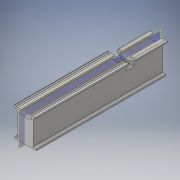
# Autodesk Inventor part: BED
Saved by Autodesk Inventor 2016 (Build 200138000, 138)
## iProperties
Created: 2017-02-14
Part Number: BED
Material: Generic
Document SubType Name: Modeling
Designer: M228540
Density: 1 g/cm^3
Appearance: Default
Author: M228540
Autodesk Inventor part; units mm, degrees
ref_plane "YZ Plane" through (0, 0, 0) normal (1, 0, 0) x (0, 1, 0)
ref_plane "XZ Plane" through (0, 0, 0) normal (0, 1, 0) x (-1, 0, 0)
ref_plane "XY Plane" through (0, 0, 0) normal (0, 0, 1) x (1, 0, 0)
sketch "Sketch1" plane through (0, 0, 0) normal (0, 0, 1) x (1, 0, 0)
  line L0 (11.5953, 6.0815) -> (2.069, 11.5815)
  line L1 (11.5953, 6.0815) -> (22.5953, 6.0815) construction
  line L2 (2.069, 11.5815) -> (-7.931, 11.5815)
  line L3 (-7.931, 11.5815) -> (-7.931, 23.2815)
  line L4 (-7.931, 23.2815) -> (0.1681, 32.9336)
  line L5 (0.1681, 32.9336) -> (3.9681, 32.9336)
  line L6 (3.9681, 32.9336) -> (11.7818, 26.3772)
  line L7 (11.7818, 26.3772) -> (11.7818, 23.1772)
  line L8 (11.7818, 23.1772) -> (27.8818, 23.1772)
  line L9 (27.8818, 23.1772) -> (27.8818, 25.1772)
  line L10 (27.8818, 25.1772) -> (53.0818, 25.1772)
  line L11 (53.0818, 25.1772) -> (53.0818, 9.4772)
  line L12 (53.0818, 9.4772) -> (38.3818, 9.4772)
  line L13 (38.3818, 9.4772) -> (38.3818, 1.4772) construction
  line L14 (38.3818, 1.4772) -> (33.763, 1.4772) construction
  line L15 (38.3818, 9.4772) -> (33.763, 1.4772)
  line L16 (38.3818, 9.4772) -> (62.019, 9.4772) construction
  line L17 (33.763, 1.4772) -> (33.763, -2.5228) construction
  arc A0 (33.763, 1.4772) -> (29.763, -2.5228) centre (33.763, -2.5228) ccw
  line L18 (29.763, -2.5228) -> (29.763, -64.5228)
  line L19 (29.763, -64.5228) -> (29.763, -268.5228)
  line L20 (-7.931, 11.5815) -> (84.2692, 11.5815) construction
  line L21 (-100.1266, 12.4772) -> (-100.1425, 25.1772)
  line L22 (-100.1425, 25.1772) -> (-136.3425, 25.1772)
  line L23 (-100.1425, 25.1772) -> (-63.9425, 25.1772) construction
  line L24 (-136.3425, 25.1772) -> (-136.3425, 23.1772)
  line L25 (-136.3425, 23.1772) -> (-155.3425, 23.1772)
  line L26 (-155.3425, 23.1772) -> (-155.3449, 25.1772)
  line L27 (-155.3449, 25.1772) -> (-163.8415, 35.279)
  line L28 (-163.8415, 35.279) -> (-168.4415, 35.279)
  line L29 (-168.4415, 35.279) -> (-180.6862, 24.9801)
  line L30 (-180.6862, 24.9801) -> (-180.6862, 10.9801)
  line L31 (-180.6862, 10.9801) -> (-166.6862, 10.9801)
  line L32 (-166.6862, 10.9801) -> (-166.6862, 7.9801) construction
  line L33 (-166.6862, 7.9801) -> (-164.9541, 7.9801) construction
  line L34 (-166.6862, 10.9801) -> (-164.9541, 7.9801)
  line L35 (-166.6862, 10.9801) -> (-161.6857, 10.9801) construction
  line L36 (-164.9541, 7.9801) -> (-146.5541, 7.9801)
  line L37 (-146.5541, 7.9801) -> (-146.5541, -14.5199)
  line L38 (-146.5541, -14.5199) -> (-146.5541, -24.0199) construction
  arc A1 (-137.0541, -24.0199) -> (-146.5541, -14.5199) centre (-146.5541, -24.0199) ccw
  line L39 (-137.0541, -24.0199) -> (-137.0541, -170.0199)
  line L40 (-137.0541, -24.0199) -> (8.9459, -24.0199) construction
  line L41 (-137.0541, -170.0199) -> (-146.5541, -170.0199)
  line L42 (-146.5541, -170.0199) -> (-146.5541, -225.5199)
  line L43 (-146.5541, -225.5199) -> (-137.0541, -225.5228)
  line L44 (-137.0541, -225.5228) -> (-137.0671, -268.5228)
  line L45 (-137.0541, -24.0199) -> (-146.5541, -24.0199) construction
  line L46 (29.763, -2.5228) -> (33.763, -2.5228) construction
  line L47 (-137.0671, -268.5228) -> (-172.0671, -268.5228)
  line L48 (-137.0671, -268.5228) -> (-102.0671, -268.5228) construction
  line L49 (-172.0671, -268.5228) -> (-172.0671, -286.5228)
  line L50 (29.763, -268.5228) -> (64.763, -268.5228)
  line L51 (29.763, -268.5228) -> (64.763, -268.5228) construction
  line L52 (64.763, -268.5228) -> (64.763, -286.5228)
  line L53 (64.763, -286.5228) -> (-172.0671, -286.5228)
  line L54 (-100.1266, 12.4772) -> (-110.7266, 12.4772)
  line L55 (-100.1266, 12.4772) -> (-89.5266, 12.4772) construction
  line L56 (-110.7266, 12.4772) -> (-114.7266, 5.549)
  line L57 (-114.7266, 5.549) -> (-119.5671, 2.9756) construction
  line L58 (-119.5671, 2.9756) -> (-124.3705, -2.5228) construction
  line L59 (-124.3705, -2.5228) -> (-125.2548, -12.6863) construction
  line L60 (-125.2548, -12.6863) -> (-112.7266, -22.8361) construction
  line L61 (-112.7266, -22.8361) -> (-52.4666, -29.0664) construction
  line L62 (-52.4666, -29.0664) -> (0.1681, -24.0199) construction
  line L63 (0.1681, -24.0199) -> (13.3927, -17.3024) construction
  line L64 (13.3927, -17.3024) -> (19.8318, -6.1886) construction
  line L65 (19.8318, -6.1886) -> (14.7109, 4.2827) construction
  line L66 (14.7109, 4.2827) -> (11.5953, 6.0815) construction
  spline S0 degree 4 poles (-114.7266, 5.549) (-119.5671, 2.9756) (-124.3705, -2.5228) (-125.2548, -12.6863) (-112.7266, -22.8361) (-52.4666, -29.0664) (0.1681, -24.0199) (13.3927, -17.3024) (19.8318, -6.1886) (14.7109, 4.2827) (11.5953, 6.0815) knots 0 0 0 0 0 1 2 3 4 5 6 7 7 7 7 7
  point P0 (0, 0)
  dimension "d0" = 11
  dimension "d1" = 150
  dimension "d2" = 10
  dimension "d3" = 11.7
  dimension "d4" = 12.6
  dimension "d5" = 140
  dimension "d6" = 3.8
  dimension "d7" = 10.2
  dimension "d8" = 140
  dimension "d9" = 3.2
  dimension "d10" = 16.1
  dimension "d11" = 2
  dimension "d12" = 25.2
  dimension "d13" = 15.7
  dimension "d14" = 14.7
  dimension "d15" = 8
  dimension "d16" = 120
  dimension "d17" = 4
  dimension "d18" = 62
  dimension "d19" = 204
  dimension "d22" = 92.2
  dimension "d24" = 12.7
  dimension "d25" = 36.2
  dimension "d26" = 180
  dimension "d27" = 2
  dimension "d28" = 19
  dimension "d29" = 2
  dimension "d30" = 13.2
  dimension "d31" = 140
  dimension "d32" = 4.6
  dimension "d33" = 16
  dimension "d34" = 139.933
  dimension "d35" = 14
  dimension "d36" = 14
  dimension "d37" = 90
  dimension "d38" = 3
  dimension "d39" = 60
  dimension "d40" = 18.4
  dimension "d41" = 22.5
  dimension "d42" = 9.5
  dimension "d43" = 146
  dimension "d44" = 90
  dimension "d45" = 9.5
  dimension "d46" = 55.5
  dimension "d47" = 90
  dimension "d48" = 9.5
  dimension "d49" = 43
  dimension "d50" = 90
  dimension "d51" = 35
  dimension "d52" = 180
  dimension "d53" = 18
  dimension "d54" = 90
  dimension "d55" = 35
  dimension "d57" = 18
  dimension "d58" = 10.6
  dimension "d59" = 180
  dimension "d60" = 8
  dimension "d61" = 120
  dimension "d62" = 62
  constraints: 114 end point, 21 perpendicular, 19 horizontal, 6 equal length, 5 vertical, 4 point on circle, 4 point on line, 2 centre point, 2 coincident, 2 parallel, 1 collinear, 3 other
  measures "d0" distance of L0.start L0.end
  measures "d1" angle of L1 L0
  measures "d2" distance of L0.end L2.end
  measures "d3" distance of L2.end L3.end
  measures "d4" distance of L3.end L4.end
  measures "d5" angle of L3 L4
  measures "d6" distance of L4.end L5.end
  measures "d7" distance of L5.end L6.end
  measures "d8" angle of L5 L6
  measures "d9" distance of L6.end L7.end
  measures "d10" distance of L7.end L8.end
  measures "d11" distance of L8.end L9.end
  measures "d12" distance of L9.end L10.end
  measures "d13" distance of L10.end L11.end
  measures "d14" distance of L11.end L12.end
  measures "d15" distance of L12.end L13.end
  measures "d16" angle of L15 L16
  measures "d17" distance of L14.end L17.end
  measures "d18" distance of L18.start L18.end
  measures "d19" distance of L18.end L19.end
  measures "d22" distance of L2.end L21.start
  measures "d24" distance of L21.start L21.end
  measures "d25" distance of L21.end L22.end
  measures "d26" angle of L22 L23
  measures "d27" distance of L22.end L24.end
  measures "d28" distance of L24.end L25.end
  measures "d29" distance of L25.end L26.end
  measures "d30" distance of L26.end L27.end
  measures "d31" angle of L27 L26
  measures "d32" distance of L27.end L28.end
  measures "d33" distance of L28.end L29.end
  measures "d34" angle of L29 L28
  measures "d35" distance of L29.end L30.end
  measures "d36" distance of L30.end L31.end
  measures "d37" angle of L31 L30
  measures "d38" distance of L31.end L32.end
  measures "d39" angle of L34 L35
  measures "d40" distance of L33.end L36.end
  measures "d41" distance of L36.end L37.end
  measures "d42" distance of L37.end L38.end
  measures "d43" distance of L39.start L39.end
  measures "d44" angle of L39 L40
  measures "d45" distance of L39.end L41.end
  measures "d46" distance of L41.end L42.end
  measures "d47" angle of L42 L41
  measures "d48" distance of L42.end L43.end
  measures "d49" distance of L43.end L44.end
  measures "d50" angle of L43 L44
  measures "d51" distance of L44.end L47.end
  measures "d52" angle of L47 L48
  measures "d53" distance of L47.end L49.end
  measures "d54" angle of L49 L47
  measures "d55" distance of L19.end L50.end
  measures "d57" distance of L50.end L52.end
  measures "d58" distance of L21.start L54.end
  measures "d59" angle of L54 L55
  measures "d60" distance of L54.end L56.end
  measures "d61" angle of L56 L54
  measures "d62" distance from line of L5 L61.end
extrude "Extrusion1" add sketch "Sketch1" against normal blind 1420
chamfer "Chamfer1" distance 9 angle 45 2 edges at (-137.0541, -170.0199, -710) (-137.0541, -225.5228, -710)
ref_plane "Work Plane3" through (-63.8022, 24.9801, -1420) normal (-1, 0, 0) x (0, 0, 1)
sketch "Sketch2" plane through (-63.8022, 24.9801, -1420) normal (-1, 0, 0) x (0, 0, 1)
  line L0 (1420, 7.9536) -> (0, 7.9536) projected
  line L1 (400, 7.9536) -> (400, -79.7464)
  line L2 (400, -79.7464) -> (318, -79.7464)
  line L3 (318, -79.7464) -> (318, 139.9786)
  line L4 (1420, -27.5029) -> (0, -27.5029) projected
  line L5 (318, 139.9786) -> (400, 139.9786)
  line L6 (400, 139.9786) -> (400, 7.9536)
  line L7 (1420, -27.5029) -> (1420, -293.5029) projected
  point P0 (1420, -24.9801)
  dimension "d68" = 1020
  dimension "d69" = 82
  dimension "d70" = 87.7
  constraints: 10 end point, 4 perpendicular, 2 point on line, 1 vertical
  measures "d68" distance between parallel lines of L7 L1
  measures "d69" distance of L1.end L2.end
  measures "d70" distance between parallel lines of L2 L0
extrude "Extrusion2" cut sketch "Sketch2" along normal through all both and the other way through all
sketch "Sketch3" plane through (0, 0, -1420) normal (0, 0, -1) x (-1, 0, 0)
  line L0 (-11.7818, 23.1772) -> (13.8436, 23.1772)
  line L1 (13.8436, 23.1772) -> (13.8436, 36.4508)
  line L2 (13.8436, 36.4508) -> (-11.7818, 36.4508)
  line L3 (-11.7818, 26.3772) -> (-11.7818, 23.1772) projected
  line L4 (-11.7818, 36.4508) -> (-11.7818, 23.1772)
  point P0 (0, 0)
  constraints: 8 end point, 2 perpendicular, 1 collinear, 1 horizontal
extrude "Extrusion3" cut sketch "Sketch3" against normal up to surface (318 mm away)
sketch "Sketch4" plane through (0, 0, -1420) normal (0, 0, -1) x (-1, 0, 0)
  line L0 (164.9541, 7.9801) -> (146.5541, 7.9801) projected
  line L1 (146.5541, 7.9801) -> (146.5541, 39.5835)
  line L2 (146.5541, 39.5835) -> (191.2081, 39.5835)
  line L3 (191.2081, 39.5835) -> (191.2081, 7.9801)
  line L4 (191.2081, 7.9801) -> (146.5541, 7.9801)
  point P0 (0, 0)
  constraints: 8 end point, 2 perpendicular, 1 collinear, 1 vertical
extrude "Extrusion4" cut sketch "Sketch4" against normal up to surface (318 mm away)
sketch "Sketch5" plane through (0, 0, -1420) normal (0, 0, -1) x (-1, 0, 0)
  arc A0 (146.5541, -14.5199) -> (137.0541, -24.0199) centre (146.5541, -24.0199) ccw projected
  line L0 (141.9124, -15.7311) -> (133.5413, -20.3219) construction
  line L1 (133.5413, -20.3219) -> (127.2902, -24.0199) construction
  line L2 (127.2902, -24.0199) -> (113.4947, -36.7041) construction
  line L3 (113.4947, -36.7041) -> (106.0541, -58.5199) construction
  line L4 (106.0541, -58.5199) -> (109.2931, -80.2819) construction
  line L5 (109.2931, -80.2819) -> (114.3087, -116.227) construction
  line L6 (114.3087, -116.227) -> (137.0457, -197.5228) construction
  spline S0 degree 4 poles (141.9124, -15.7311) (133.5413, -20.3219) (127.2902, -24.0199) (113.4947, -36.7041) (106.0541, -58.5199) (109.2931, -80.2819) (114.3087, -116.227) (137.0457, -197.5228) knots 1 1 1 1 1 2 3 4 5 5 5 5 5
  line L7 (172.0671, -268.5228) -> (137.0671, -268.5228) projected
  line L8 (137.0541, -161.0199) -> (137.0541, -24.0199) projected
  line L9 (137.0671, -268.5228) -> (137.0568, -234.5228) projected
  line L10 (137.0457, -197.5228) -> (137.0568, -234.5228)
  line L11 (137.0568, -234.5228) -> (163.0138, -234.515)
  line L12 (163.0138, -234.515) -> (148.1613, -15.3077)
  line L13 (148.1613, -15.3077) -> (141.9124, -15.7311)
  point P0 (0, 0)
  dimension "d77" = 71
  dimension "d78" = 31
  dimension "d79" = 44
  constraints: 8 end point, 2 perpendicular, 1 collinear, 1 point on circle, 3 other
  measures "d77" distance from line of L7 L6.end
  measures "d78" distance from line of L8 L3.end
  measures "d79" vertical distance of A0.start L3.end
extrude "Extrusion5" cut sketch "Sketch5" against normal up to surface (318 mm away)
sketch "Sketch6" plane through (0, 0, -1420) normal (0, 0, -1) x (-1, 0, 0)
  line L0 (146.5541, 23.1772) -> (136.3425, 23.1772) projected
  line L1 (136.3425, 23.1772) -> (136.3425, 25.1772) projected
  line L2 (136.3425, 25.1772) -> (100.1425, 25.1772) projected
  line L3 (100.1425, 25.1772) -> (100.1266, 12.4772) projected
  line L4 (100.1266, 12.4772) -> (110.7266, 12.4772) projected
  line L5 (110.7266, 12.4772) -> (114.7266, 5.549) projected
  spline S0 degree 4 poles (114.7266, 5.549) (119.5671, 2.9756) (124.3705, -2.5228) (125.2548, -12.6863) (112.7266, -22.8361) (52.4666, -29.0664) (-0.1681, -24.0199) (-13.3927, -17.3024) (-19.8318, -6.1886) (-14.7109, 4.2827) (-11.5953, 6.0815) knots 0 0 0 0 0 0.142857 0.285714 0.428571 0.571429 0.714286 0.857143 1 1 1 1 1 projected
  line L6 (146.5541, -14.5199) -> (146.5541, 23.1772) projected
  line L7 (-11.5953, 6.0815) -> (-2.069, 11.5815) projected
  line L8 (-2.069, 11.5815) -> (7.931, 11.5815) projected
  line L9 (7.931, 11.5815) -> (7.931, 23.1772) projected
  line L10 (7.931, 23.1772) -> (-27.8818, 23.1772) projected
  line L11 (-27.8818, 25.1772) -> (-53.0818, 25.1772) projected
  line L12 (-27.8818, 23.1772) -> (-27.8818, 25.1772) projected
  line L13 (-53.0818, 25.1772) -> (-53.0818, 9.4772) projected
  line L14 (-53.0818, 9.4772) -> (-38.3818, 9.4772) projected
  line L15 (-38.3818, 9.4772) -> (-33.763, 1.4772) projected
  arc A0 (-29.763, -2.5228) -> (-33.763, 1.4772) centre (-33.763, -2.5228) ccw projected
  line L16 (-33.763, 1.4772) -> (-15.3871, 1.4772)
  line L17 (120.2323, 1.4772) -> (146.5541, 1.4772)
  point P0 (0, 0)
  constraints: 4 end point, 2 perpendicular, 2 tangent, 1 point on line, 3 other
extrude "Extrusion6" add sketch "Sketch6" along normal blind 26
body "Solid1"
